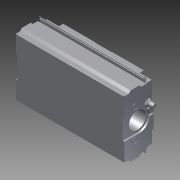
# Autodesk Inventor part: KR55(A-1)-Slider
Saved by Autodesk Inventor 2011 SP1 (Build 150282100, 282)
## iProperties
Created: 2013-10-23
Part Number: KR55(A-1)-Slider
Catalog Web Link: www.cadenas.de
Description: LM Guide Actuator - Slider-KR
Vendor: THK
Document SubType Name: Modeling
Designer: PARTuser1
Manufacturer: THK
Density: 1 g/cm^3
Category: PARTsolutions
Company: THK
Title: KR55(A-1)-Slider
Author: Cadenas PARTsolutions
Comments: KR
PSOL_IDENT_0: {$CADENAS_DATA\23d-libs\thk\lm_guide_actuator\type_kr\parts\lm_g_a_kr_slider.prj},201 {VTYP=3D},{NB=
PSOL_IDENT_1: KR55(A-1)-Slider},{LINA=KR55(A-1)-Slider},{NN=LM Guide Actuator - Slider},{DATE=20.05.2010 07:50:26}
PSOL_IDENT_2: ,{GEOMDATE=20.05.2010 07:49:00},{VERSION=},{LINEID=80},{LINESUBID=-1},{WBVAR=TNB,POS}  {NB=KR55(A-1)
PSOL_IDENT_3: -Slider},{LINA=KR55(A-1)-Slider},{KT=DUMMY},{ORDER=KR55},{XTYPE=8.000},{TNB=A},{L=128},{TNB1='A','B'
PSOL_IDENT_4: },{POS=1}
CNS_NT: KR
CNS_NB: KR55(A-1)-Slider
CNS_NBSYN: $ORDER.($TNB.-$POS.)-Slider
CNS_LINA: KR55(A-1)-Slider
CNS_ORDER: KR55
CNS_XTYPE: 8.000
CNS_TNB: A
CNS_L: 128.000
CNS_TNB1: 'A','B'
CNS_POS: 1
SUPPLIER: THK
ARTICLENO: KR55(A-1)-Slider
BOMINFO: KR55(A-1)-Slider
CREATOR: CADENAS GmbH
Autodesk Inventor part; units mm, degrees
sketch "Sketch_1" plane through (0, 0, 0) normal (1, 0, 0) x (0, 1, 0)
  line L0 (8.229, 39.991) -> (8.0169, 39.7789)
  line L1 (8.0169, 39.7789) -> (8.98, 38.4034)
  line L2 (8.98, 38.4034) -> (8.98, 37.8)
  line L3 (8.98, 37.8) -> (8.58, 37.4)
  line L4 (8.58, 37.4) -> (8.58, 33.87)
  line L5 (8.58, 33.87) -> (2.5, 33.87)
  line L6 (2.5, 33.87) -> (0.07, 36.3)
  line L7 (0.07, 36.3) -> (-10.07, 36.3)
  line L8 (-10.07, 36.3) -> (-12.5, 33.87)
  line L9 (-12.5, 33.87) -> (-17.33, 33.87)
  line L10 (-17.33, 33.87) -> (-17.6, 33.6)
  line L11 (-17.6, 33.6) -> (-17.6, -33.6)
  line L12 (-17.6, -33.6) -> (-17.33, -33.87)
  line L13 (-17.33, -33.87) -> (-12.5, -33.87)
  line L14 (-12.5, -33.87) -> (-10.07, -36.3)
  line L15 (-10.07, -36.3) -> (0.07, -36.3)
  line L16 (0.07, -36.3) -> (2.5, -33.87)
  line L17 (2.5, -33.87) -> (8.58, -33.87)
  line L18 (8.58, -33.87) -> (8.58, -37.4)
  line L19 (8.58, -37.4) -> (8.98, -37.8)
  line L20 (8.98, -37.8) -> (8.98, -38.4034)
  line L21 (8.98, -38.4034) -> (8.0169, -39.7789)
  line L22 (8.0169, -39.7789) -> (8.229, -39.991)
  line L23 (8.229, -39.991) -> (9.82, -38.4)
  line L24 (9.82, -38.4) -> (9.82, -35.9)
  line L25 (9.82, -35.9) -> (9.58, -35.9)
  line L26 (9.58, -35.9) -> (9.58, -32.9)
  line L27 (9.58, -32.9) -> (8.58, -32.9)
  line L28 (8.58, -32.9) -> (8.58, -32.5)
  line L29 (8.58, -32.5) -> (17, -32.5)
  line L30 (17, -32.5) -> (17, 32.5)
  line L31 (17, 32.5) -> (8.58, 32.5)
  line L32 (8.58, 32.5) -> (8.58, 32.9)
  line L33 (8.58, 32.9) -> (9.58, 32.9)
  line L34 (9.58, 32.9) -> (9.58, 35.9)
  line L35 (9.58, 35.9) -> (9.82, 35.9)
  line L36 (9.82, 35.9) -> (9.82, 38.4)
  line L37 (9.82, 38.4) -> (8.229, 39.991)
  circle A0 centre (0, 0) radius 10
  constraints: 76 end point, 1 centre point
extrude "Extrusion1" add sketch "Sketch_1" along normal mid plane 124
sketch "Sketch_2" plane through (62, 0, 0) normal (1, 0, 0) x (0, 0, -1)
  line L0 (-36.29, 0.06) -> (-36.29, -10.07)
  line L1 (-36.29, -10.07) -> (-33.86, -12.5)
  line L2 (-33.86, -12.5) -> (-33.86, -17.33)
  line L3 (-33.86, -17.33) -> (-33.78, -17.41)
  line L4 (-33.78, -17.41) -> (-12.5, -17.41)
  line L5 (-12.5, -17.41) -> (-12.5, 0)
  arc A0 (-1, 12.4599) -> (-12.5, 0) centre (0, 0) ccw
  line L6 (-1, 12.4599) -> (-1, 16.99)
  line L7 (-1, 16.99) -> (-15.79, 16.99)
  line L8 (-15.79, 16.99) -> (-16.79, 15.99)
  line L9 (-16.79, 15.99) -> (-16.79, 9.99)
  line L10 (-16.79, 9.99) -> (-31.29, 9.99)
  line L11 (-31.29, 9.99) -> (-32.29, 8.99)
  line L12 (-32.29, 8.99) -> (-32.29, 8.49)
  line L13 (-32.29, 8.49) -> (-33.86, 8.49)
  line L14 (-33.86, 8.49) -> (-33.86, 2.49)
  line L15 (-33.86, 2.49) -> (-36.29, 0.06)
  constraints: 32 end point, 2 point on circle, 1 centre point
extrude "Extrusion2" add sketch "Sketch_2" along normal blind 2
sketch "Sketch_3" plane through (62, 0, 0) normal (1, 0, 0) x (0, 0, -1)
  arc A0 (12.5, 0) -> (1, 12.4599) centre (0, 0) ccw
  line L0 (12.5, 0) -> (12.5, -17.41)
  line L1 (12.5, -17.41) -> (33.78, -17.41)
  line L2 (33.78, -17.41) -> (33.86, -17.33)
  line L3 (33.86, -17.33) -> (33.86, -12.5)
  line L4 (33.86, -12.5) -> (36.29, -10.07)
  line L5 (36.29, -10.07) -> (36.29, 0.06)
  line L6 (36.29, 0.06) -> (33.86, 2.49)
  line L7 (33.86, 2.49) -> (33.86, 8.49)
  line L8 (33.86, 8.49) -> (32.29, 8.49)
  line L9 (32.29, 8.49) -> (32.29, 8.99)
  line L10 (32.29, 8.99) -> (31.29, 9.99)
  line L11 (31.29, 9.99) -> (16.79, 9.99)
  line L12 (16.79, 9.99) -> (16.79, 15.99)
  line L13 (16.79, 15.99) -> (15.79, 16.99)
  line L14 (15.79, 16.99) -> (1, 16.99)
  line L15 (1, 16.99) -> (1, 12.4599)
  constraints: 32 end point, 2 point on circle, 1 centre point
extrude "Extrusion3" add sketch "Sketch_3" along normal blind 2
sketch "Sketch_4" plane through (-62, 0, 0) normal (1, 0, 0) x (0, 0, -1)
  line L0 (-36.29, 0.06) -> (-36.29, -10.07)
  line L1 (-36.29, -10.07) -> (-33.86, -12.5)
  line L2 (-33.86, -12.5) -> (-33.86, -17.33)
  line L3 (-33.86, -17.33) -> (-33.78, -17.41)
  line L4 (-33.78, -17.41) -> (-12.5, -17.41)
  line L5 (-12.5, -17.41) -> (-12.5, 0)
  arc A0 (-1, 12.4599) -> (-12.5, 0) centre (0, 0) ccw
  line L6 (-1, 12.4599) -> (-1, 16.99)
  line L7 (-1, 16.99) -> (-15.79, 16.99)
  line L8 (-15.79, 16.99) -> (-16.79, 15.99)
  line L9 (-16.79, 15.99) -> (-16.79, 9.99)
  line L10 (-16.79, 9.99) -> (-31.29, 9.99)
  line L11 (-31.29, 9.99) -> (-32.29, 8.99)
  line L12 (-32.29, 8.99) -> (-32.29, 8.49)
  line L13 (-32.29, 8.49) -> (-33.86, 8.49)
  line L14 (-33.86, 8.49) -> (-33.86, 2.49)
  line L15 (-33.86, 2.49) -> (-36.29, 0.06)
  constraints: 32 end point, 2 point on circle, 1 centre point
extrude "Extrusion4" add sketch "Sketch_4" against normal blind 2
sketch "Sketch_5" plane through (-62, 0, 0) normal (1, 0, 0) x (0, 0, -1)
  arc A0 (12.5, 0) -> (1, 12.4599) centre (0, 0) ccw
  line L0 (12.5, 0) -> (12.5, -17.41)
  line L1 (12.5, -17.41) -> (33.78, -17.41)
  line L2 (33.78, -17.41) -> (33.86, -17.33)
  line L3 (33.86, -17.33) -> (33.86, -12.5)
  line L4 (33.86, -12.5) -> (36.29, -10.07)
  line L5 (36.29, -10.07) -> (36.29, 0.06)
  line L6 (36.29, 0.06) -> (33.86, 2.49)
  line L7 (33.86, 2.49) -> (33.86, 8.49)
  line L8 (33.86, 8.49) -> (32.29, 8.49)
  line L9 (32.29, 8.49) -> (32.29, 8.99)
  line L10 (32.29, 8.99) -> (31.29, 9.99)
  line L11 (31.29, 9.99) -> (16.79, 9.99)
  line L12 (16.79, 9.99) -> (16.79, 15.99)
  line L13 (16.79, 15.99) -> (15.79, 16.99)
  line L14 (15.79, 16.99) -> (1, 16.99)
  line L15 (1, 16.99) -> (1, 12.4599)
  constraints: 32 end point, 2 point on circle, 1 centre point
extrude "Extrusion5" add sketch "Sketch_5" against normal blind 2
sketch "Sketch_8" plane through (0, 0, 0) normal (1, 0, 0) x (0, 1, 0)
  line L0 (17, 32.5) -> (17, -32.5)
  line L1 (17, -32.5) -> (22, -32.5)
  line L2 (22, -32.5) -> (23, -31.5)
  line L3 (23, -31.5) -> (23, -16.8)
  line L4 (23, -16.8) -> (21.2, -15)
  line L5 (21.2, -15) -> (21.2, 15)
  line L6 (21.2, 15) -> (23, 16.8)
  line L7 (23, 16.8) -> (23, 31.5)
  line L8 (23, 31.5) -> (22, 32.5)
  line L9 (22, 32.5) -> (17, 32.5)
  constraints: 20 end point
extrude "Extrusion6" add sketch "Sketch_8" along normal mid plane 95.2
sketch "Sketch_9" plane through (0, 0, 0) normal (1, 0, 0) x (0, 0, -1)
  line L0 (-35, 21.6) -> (35, 21.6)
  line L1 (35, 21.6) -> (35, 31.6)
  line L2 (35, 31.6) -> (-35, 31.6)
  line L3 (-35, 31.6) -> (-35, 21.6)
  constraints: 8 end point
extrude "Extrusion7" cut sketch "Sketch_9" along normal mid plane 20
sketch "Sketch_11" plane through (0, -5, 0) normal (0, 1, 0) x (1, 0, 0)
  line L0 (65, 17) -> (62.5, 17)
  line L1 (62.5, 19.75) -> (65, 19.75)
  line L2 (65, 19.75) -> (65, 20.05)
  line L3 (65, 20.05) -> (62.5, 20.05)
  line L4 (62.5, 20.05) -> (62.5, 19.75)
  constraints: 10 end point
revolve "Revolution1" cut sketch "Sketch_11" angle 360 about axis through (65, -5, -17) along (1, 0, 0)
sketch "Sketch_12" plane through (0, -5, 0) normal (0, 1, 0) x (1, 0, 0)
  line L0 (65, -17) -> (62.5, -17)
  line L1 (62.5, -14.25) -> (65, -14.25)
  line L2 (65, -14.25) -> (65, -13.95)
  line L3 (65, -13.95) -> (62.5, -13.95)
  line L4 (62.5, -13.95) -> (62.5, -14.25)
  constraints: 10 end point
revolve "Revolution2" cut sketch "Sketch_12" angle 360 about axis through (65, -5, 17) along (1, 0, 0)
sketch "Sketch_13" plane through (0, -5, 0) normal (0, 1, 0) x (1, 0, 0)
  line L0 (-62.5, 17) -> (-65, 17)
  line L1 (-65, 19.75) -> (-62.5, 19.75)
  line L2 (-62.5, 19.75) -> (-62.5, 20.05)
  line L3 (-62.5, 20.05) -> (-65, 20.05)
  line L4 (-65, 20.05) -> (-65, 19.75)
  constraints: 10 end point
revolve "Revolution3" cut sketch "Sketch_13" angle 360 about axis through (-62.5, -5, -17) along (1, 0, 0)
sketch "Sketch_14" plane through (0, -5, 0) normal (0, 1, 0) x (1, 0, 0)
  line L0 (-62.5, -17) -> (-65, -17)
  line L1 (-65, -14.25) -> (-62.5, -14.25)
  line L2 (-62.5, -14.25) -> (-62.5, -13.95)
  line L3 (-62.5, -13.95) -> (-65, -13.95)
  line L4 (-65, -13.95) -> (-65, -14.25)
  constraints: 10 end point
revolve "Revolution4" cut sketch "Sketch_14" angle 360 about axis through (-62.5, -5, 17) along (1, 0, 0)
sketch "Sketch12" plane through (47.6, 23, -16.8) normal (0, 1, 0) x (1, 0, 0)
  point P0 (-22.6, 8.2)
hole "Drilling 1" at (25, 23, -25) direction (0, -1, 0) diameter 6.647 depth 16 tip angle 140 countersink diameter 8 countersink angle 90 thread size "M8x1.25" class "6H" standard "ISO Metric profile"
pattern_linear "Rectangular Pattern1" count 2 spacing 50 along (-1, 0, 0) count 2 spacing 50 along (0, 0, 1) of "Drilling 1"
sketch "Sketch13" plane through (-10, 21.6, -32.5) normal (0, 1, 0) x (1, 0, 0)
  point P0 (6, -7.5)
hole "Drilling 2" at (-4, 21.6, -25) direction (0, -1, 0) diameter 2.459 depth 7 tip angle 140 countersink diameter 3 countersink angle 90 thread size "M3x0.5" class "6H" standard "ISO Metric profile"
pattern_linear "Rectangular Pattern2" count 2 spacing 8 along (1, 0, 0) count 2 spacing 50 along (0, 0, 1) of "Drilling 2"
sketch "Sketch_17" plane through (0, 12, 0) normal (0, 1, 0) x (1, 0, 0)
  line L0 (62, -12) -> (70.6, -12)
  arc A0 (70.1, -13.245) -> (70.6, -12) centre (68.8, -12) ccw
  line L1 (70.1, -13.245) -> (70.1, -14.4)
  line L2 (70.1, -14.4) -> (67.4, -15.3)
  line L3 (67.4, -15.3) -> (66.0758, -14.8616)
  arc A1 (66.0758, -14.8616) -> (65.2615, -14.9449) centre (65.7615, -15.8109) ccw
  line L4 (65.2615, -14.9449) -> (64.3, -15.5)
  line L5 (64.3, -15.5) -> (64.0452, -16.2)
  line L6 (64.0452, -16.2) -> (62.2548, -16.2)
  line L7 (62.2548, -16.2) -> (62, -15.5)
  line L8 (62, -15.5) -> (62, -12)
  line L9 (62, -12) -> (70.6, -12)
  constraints: 20 end point, 4 point on circle, 2 centre point
revolve "Revolution5" add sketch "Sketch_17" angle 360 about axis through (62, 12, 12) along (-1, 0, 0)
sketch "Sketch_18" plane through (64, 0, 0) normal (1, 0, 0) x (0, 0, -1)
  line L0 (-17, 6) -> (-7, 6)
  line L1 (-7, 6) -> (-7, 18)
  line L2 (-7, 18) -> (-17, 18)
  line L3 (-17, 18) -> (-17, 6)
  line L4 (-15.5, 14.0207) -> (-15.5, 9.9793)
  line L5 (-15.5, 9.9793) -> (-12, 7.9585)
  line L6 (-12, 7.9585) -> (-8.5, 9.9793)
  line L7 (-8.5, 9.9793) -> (-8.5, 14.0207)
  line L8 (-8.5, 14.0207) -> (-12, 16.0415)
  line L9 (-12, 16.0415) -> (-15.5, 14.0207)
  constraints: 20 end point
extrude "Extrusion8" cut sketch "Sketch_18" along normal mid plane 4
ref_plane "slider_body_XY" through (0, 0, 0) normal (1, 0, 0) x (0, 0, -1)
ref_plane "slider_body_YZ" through (0, 0, 0) normal (0, 0, -1) x (0, 1, 0)
ref_plane "slider_body_ZX" through (0, 0, 0) normal (0, 1, 0) x (1, 0, 0)
ref_plane "slider_sensor_dog_XY" through (0, 21.6, 25) normal (0, 1, 0) x (1, 0, 0)
ref_plane "slider_sensor_dog_YZ" through (0, 21.6, 25) normal (1, 0, 0) x (0, 0, -1)
ref_plane "slider_sensor_dog_ZX" through (0, 21.6, 25) normal (0, 0, -1) x (0, 1, 0)
ref_plane "slider_slider_spacer_XY" through (0, 23, 0) normal (0, 1, 0) x (1, 0, 0)
ref_plane "slider_slider_spacer_YZ" through (0, 23, 0) normal (1, 0, 0) x (0, 0, -1)
ref_plane "slider_slider_spacer_ZX" through (0, 23, 0) normal (0, 0, -1) x (0, 1, 0)
body "Solid1"
